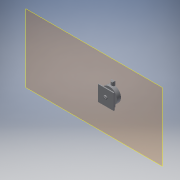
# Autodesk Inventor part: Part42
Saved by Autodesk Inventor 2016 (Build 200138000, 138)
## iProperties
Created: 2016-01-27
Part Number: Part42
Material: Generic
Document SubType Name: Modeling
Designer: seve
Density: 1 g/cm^3
Appearance: Default
Author: seve
Autodesk Inventor part; units mm, degrees
ref_plane "YZ Plane" through (0, 0, 0) normal (1, 0, 0) x (0, 1, 0)
ref_plane "XZ Plane" through (0, 0, 0) normal (0, 1, 0) x (-1, 0, 0)
ref_plane "XY Plane" through (0, 0, 0) normal (0, 0, 1) x (1, 0, 0)
ref_plane "Work Plane1" through (0, 0, 0) normal (0, 0, 1) x (1, 0, 0)
sketch "Sketch1" plane through (0, 0, 0) normal (0, 0, 1) x (1, 0, 0)
  circle A0 centre (15.5909, 3.8029) radius 6.35
  point P0 (0, 0)
  dimension "d2" = 12.7
  constraints: 1 centre point
  measures "d2" diameter of A0
extrude "Extrusion1" add sketch "Sketch1" along normal blind 3.175
sketch "Sketch2" plane through (15.5909, 3.8029, 0) normal (0, 0, -1) x (-1, 0, 0)
  line L0 (-1.6201, 9.5156) -> (1.414, 9.5156)
  line L1 (1.414, 9.5156) -> (1.414, -9.1153)
  line L2 (1.414, -9.1153) -> (-1.6201, -9.1153)
  line L3 (-1.6201, -9.1153) -> (-1.6201, 9.5156)
  point P0 (15.5909, -3.8029)
  constraints: 8 end point, 2 parallel, 1 horizontal, 1 perpendicular
extrude "Extrusion2" add sketch "Sketch2" against normal blind 1.5875
chamfer "Chamfer1" distance 0.7937 angle 45 6 edges at (15.694, 13.3185, 1.5875) (14.1769, 11.656, 1.5875) (17.211, 11.6306, 1.5875) (14.1769, -3.85, 1.5875) (15.694, -5.3124, 1.5875) (17.211, -3.8247, 1.5875)
shell "Shell1" thickness 0.508 removed faces 1 at (15.2921, 5.5449, 3.175)
sketch "Sketch3" plane through (14.6849, 12.8105, 0.508) normal (0, 0, 1) x (1, 0, 0)
  arc A0 (2.018, -14.7428) -> (2.018, -3.2724) centre (0.906, -9.0076) ccw projected
  line L0 (2.018, -3.2724) -> (2.018, 0) projected
  line L1 (2.018, 0) -> (0, 0) projected
  line L2 (0, 0) -> (0, -3.2363) projected
  arc A1 (0, -3.2363) -> (0, -14.7789) centre (0.906, -9.0076) ccw projected
  line L3 (0, -14.7789) -> (0, -17.6149) projected
  line L4 (0, -17.6149) -> (2.018, -17.6149) projected
  line L5 (2.018, -17.6149) -> (2.018, -14.7428) projected
  circle A2 centre (0.906, -9.0076) radius 5.842
  point P0 (-14.6849, -12.8105)
  constraints: 1 centre point, 1 coincident, 1 concentric
extrude "Extrusion3" add sketch "Sketch3" along normal blind 1.5875 contours A2 A1 A0
sketch "Sketch4" plane through (15.5909, 3.8029, 2.0955) normal (0, 0, 1) x (1, 0, 0)
  circle A0 centre (0, 0) radius 5.842 projected
  circle A1 centre (0, 0) radius 1.5875
  point P0 (-15.5909, -3.8029)
  dimension "d11" = 3.175
  constraints: 1 centre point, 1 coincident
  measures "d11" diameter of A1
extrude "Extrusion4" add sketch "Sketch4" along normal blind 3.175 contours A1
sketch "Sketch5" plane through (15.5909, 3.8029, 5.2705) normal (0, 0, 1) x (1, 0, 0)
  circle A0 centre (0, 0) radius 1.5875 projected
  circle A1 centre (0, 0) radius 6.35 projected
  line L0 (6.35, -6.35) -> (-6.35, -6.35)
  line L1 (-6.35, -6.35) -> (-6.35, 6.35)
  line L2 (-6.35, 6.35) -> (6.35, 6.35)
  line L3 (6.35, 6.35) -> (6.35, -6.35)
  point P0 (-15.5909, -3.8029)
  constraints: 8 end point, 2 parallel, 1 horizontal, 1 perpendicular
extrude "Extrusion5" add sketch "Sketch5" along normal blind 0.7937
sketch "Sketch6" plane through (15.5909, 3.8029, 5.2705) normal (0, 0, 1) x (1, 0, 0)
  circle A0 centre (0, 0) radius 1.5875
  point P0 (-15.5909, -3.8029)
  constraints: 1 centre point
extrude "Extrusion6" add sketch "Sketch6" along normal blind 1.5875
fillet "Fillet1" radius 0.7937 1 edges at (14.0034, 3.8029, 6.858)
sketch "Sketch7" plane through (15.5909, 3.8029, 6.858) normal (0, 0, 1) x (1, 0, 0)
  line L0 (0.863, -0.1977) -> (-0.8638, -0.1977)
  line L1 (-0.8638, -0.1977) -> (-0.8638, 0.2876)
  line L2 (-0.8638, 0.2876) -> (0.863, 0.2876)
  line L3 (0.863, 0.2876) -> (0.863, -0.1977)
  line L4 (0.258, 0.8864) -> (-0.2021, 0.8864)
  line L5 (-0.2021, 0.8864) -> (-0.2021, -0.8972)
  line L6 (-0.2021, -0.8972) -> (0.258, -0.8972)
  line L7 (0.258, -0.8972) -> (0.258, 0.8864)
  point P0 (-15.5909, -3.8029)
  constraints: 16 end point, 4 parallel, 2 horizontal, 2 perpendicular
extrude "Extrusion7" cut sketch "Sketch7" against normal blind 0.3969
chamfer "Chamfer2" distance 0.1984 angle 45 5 edges at (16.4539, 3.946, 6.8539) (16.4539, 3.7043, 6.8545) (15.6187, 2.9057, 6.8512) (14.7271, 3.8475, 6.8548) (15.6183, 4.6893, 6.8525)
body "Solid1"
